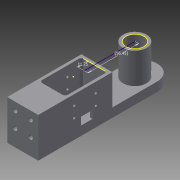
# Autodesk Inventor part: JointBase
Saved by Autodesk Inventor 2015 (Build 190159000, 159)
## iProperties
Created: 2016-04-06
Part Number: JointBase
Material: Generic
Document SubType Name: Modeling
Designer: Hatch
Density: 1 g/cm^3
Appearance: Default
Author: Hatch
Autodesk Inventor part; units mm, degrees
ref_plane "YZ Plane" through (0, 0, 0) normal (1, 0, 0) x (0, 1, 0)
ref_plane "XZ Plane" through (0, 0, 0) normal (0, 1, 0) x (-1, 0, 0)
ref_plane "XY Plane" through (0, 0, 0) normal (0, 0, 1) x (1, 0, 0)
sketch "Sketch1" plane through (0, 0, 0) normal (0, 1, 0) x (-1, 0, 0)
  line L0 (-17.25, 26.25) -> (17.25, 26.25)
  line L1 (17.25, 26.25) -> (17.25, -26.25)
  line L2 (17.25, -26.25) -> (-17.25, -26.25)
  line L3 (-17.25, -26.25) -> (-17.25, 26.25)
  line L4 (-17.25, 26.25) -> (17.25, -26.25) construction
  line L5 (17.25, 26.25) -> (-17.25, -26.25) construction
  line L6 (17.25, -26.25) -> (-17.25, -26.25)
  line L7 (-17.25, -26.25) -> (-17.25, -76.25)
  line L8 (-17.25, -76.25) -> (17.25, -76.25)
  line L9 (17.25, -76.25) -> (17.25, -26.25)
  arc A0 (-17.25, -76.25) -> (17.25, -76.25) centre (0, -76.25) ccw
  point P0 (0, 0)
  dimension "d0" = 34.5
  dimension "d1" = 52.5
  dimension "d4" = 50
  constraints: 20 end point, 4 parallel, 3 midpoint, 2 horizontal, 2 perpendicular, 2 point on circle, 1 centre point
  measures "d0" distance of L1.end L2.end
  measures "d1" distance of L0.end L1.end
  measures "d4" distance of L7.end L6.end
extrude "Floor" add sketch "Sketch1" along normal blind 10
sketch "Sketch3" plane through (0, 10, 0) normal (0, 1, 0) x (1, 0, 0)
  arc A0 (17.25, 76.25) -> (-17.25, 76.25) centre (0, 76.25) ccw
  circle A1 centre (0, 68.45) radius 10
  circle A2 centre (0, 68.45) radius 13
  line L0 (14.25, -23.25) -> (-14.25, -23.25)
  line L1 (-14.25, -23.25) -> (-14.25, 23.25)
  line L2 (-14.25, 23.25) -> (14.25, 23.25)
  line L3 (14.25, 23.25) -> (14.25, -23.25)
  line L4 (14.25, -23.25) -> (-14.25, 23.25) construction
  line L5 (-14.25, -23.25) -> (14.25, 23.25) construction
  line L6 (17.25, 26.25) -> (-17.25, 26.25)
  line L7 (-17.25, 26.25) -> (-17.25, -26.25)
  line L8 (-17.25, -26.25) -> (17.25, -26.25)
  line L9 (17.25, -26.25) -> (17.25, 26.25)
  line L10 (17.25, 26.25) -> (-17.25, -26.25) construction
  line L11 (-17.25, 26.25) -> (17.25, -26.25) construction
  line L12 (0, 23.25) -> (0, 68.45)
  point P0 (0, 0)
  dimension "d14" = 20
  dimension "d18" = 28.5
  dimension "d19" = 46.5
  dimension "d38" = 45.2
  dimension "d54" = 26
  constraints: 26 end point, 5 midpoint, 4 parallel, 3 centre point, 2 coincident, 2 horizontal, 2 perpendicular, 2 point on circle, 1 vertical
  measures "d14" diameter of A1
  measures "d18" distance of L1.end L2.end
  measures "d19" distance of L0.end L1.end
  measures "d38" distance of L12.start L12.end
  measures "d54" diameter of A2
extrude "Slots" add sketch "Sketch3" along normal blind 34
sketch "Sketch4" plane through (17.25, 0, 26.25) normal (1, 0, 0) x (0, 0, -1)
  line L0 (3, 10) -> (49.5, 10)
  line L1 (49.5, 10) -> (49.5, 44)
  line L2 (49.5, 44) -> (3, 44)
  line L3 (3, 44) -> (3, 10)
  line L4 (26.25, 10) -> (38.25, 10)
  line L5 (3, 10) -> (49.5, 10) projected
  line L6 (38.25, 10) -> (14.25, 10)
  line L7 (10.25, 33) -> (34.25, 33)
  line L8 (34.25, 33) -> (34.25, 21)
  line L9 (34.25, 21) -> (10.25, 21)
  line L10 (10.25, 21) -> (10.25, 33)
  line L11 (10.25, 33) -> (34.25, 21) construction
  line L12 (34.25, 33) -> (10.25, 21) construction
  circle A0 centre (10.25, 33) radius 1.35
  circle A1 centre (34.25, 33) radius 1.35
  circle A2 centre (34.25, 21) radius 1.35
  circle A3 centre (10.25, 21) radius 1.35
  line L13 (49.5, 10) -> (49.5, 44) projected
  line L14 (49.5, 27) -> (34.25, 27)
  line L15 (34.25, 27) -> (22.25, 27)
  point P0 (26.25, 0)
  point P1 (22.25, 27)
  dimension "d0" = 34.5
  dimension "d24" = 12
  dimension "d25" = 24
  dimension "d26" = 2.7
  dimension "d27" = 2.7
  dimension "d28" = 2.7
  dimension "d29" = 2.7
  dimension "d56" = 15.25
  dimension "d57" = 12
  constraints: 28 end point, 5 midpoint, 4 centre point, 4 coincident, 4 parallel, 3 perpendicular, 2 horizontal, 2 point on line
  measures "d24" distance of L7.end L8.end
  measures "d25" distance of L8.end L9.end
  measures "d26" diameter of A0
  measures "d27" diameter of A1
  measures "d28" diameter of A2
  measures "d29" diameter of A3
  measures "d56" distance of L14.start L14.end
  measures "d57" distance of L15.end L14.end
extrude "Screws/Sides" cut sketch "Sketch4" against normal through all contours A1 L7 L8 | L8 L7 A1 | A2 L9 L8 | L8 L9 A2 | A0 L10 L7 | L7 L10 A0 | A3 L10 L9 | L9 L10 A3
sketch "Sketch5" plane through (0, 44, 0) normal (0, 1, 0) x (1, 0, 0)
  line L0 (14.25, -21.25) -> (-14.25, -21.25)
  line L1 (-14.25, -21.25) -> (-14.25, 21.25)
  line L2 (-14.25, 21.25) -> (14.25, 21.25)
  line L3 (14.25, 21.25) -> (14.25, -21.25)
  line L4 (14.25, -21.25) -> (-14.25, 21.25) construction
  line L5 (-14.25, -21.25) -> (14.25, 21.25) construction
  line L6 (12.25, 23.25) -> (-12.25, 23.25)
  line L7 (-12.25, 23.25) -> (-12.25, -23.25)
  line L8 (-12.25, -23.25) -> (12.25, -23.25)
  line L9 (12.25, -23.25) -> (12.25, 23.25)
  line L10 (12.25, 23.25) -> (-12.25, -23.25) construction
  line L11 (-12.25, 23.25) -> (12.25, -23.25) construction
  line L12 (-12.25, 21.25) -> (-14.25, 21.25)
  line L13 (12.25, 23.25) -> (12.25, 21.25)
  line L14 (12.25, -21.25) -> (14.25, -21.25)
  line L15 (12.25, -23.25) -> (12.25, -21.25)
  line L16 (-14.25, -21.25) -> (-14.25, -23.25)
  line L17 (-14.25, -23.25) -> (-12.25, -23.25)
  line L18 (-14.25, -21.25) -> (-12.25, -23.25)
  line L19 (-14.25, -23.25) -> (-14.25, -21.25)
  line L20 (-14.25, 21.25) -> (-12.25, 23.25)
  line L21 (-14.25, 23.25) -> (-14.25, 21.25)
  line L22 (-14.25, -23.25) -> (-14.25, 23.25) projected
  line L23 (12.25, 23.25) -> (14.25, 23.25)
  line L24 (14.25, 23.25) -> (14.25, 21.25)
  line L25 (12.25, 23.25) -> (14.25, 21.25)
  line L26 (14.25, 23.25) -> (12.25, 23.25)
  line L27 (14.25, -23.25) -> (12.25, -23.25)
  line L28 (14.25, -23.25) -> (-14.25, -23.25) projected
  line L29 (14.25, -21.25) -> (12.25, -23.25)
  line L30 (14.25, -23.25) -> (14.25, -21.25)
  line L31 (14.25, 23.25) -> (14.25, -23.25) projected
  line L32 (-14.25, 23.25) -> (-12.25, 23.25)
  line L33 (14.25, 23.25) -> (-14.25, 23.25) projected
  point P0 (0, 0)
  dimension "d32" = 42.5
  dimension "d33" = 24.5
  constraints: 60 end point, 7 collinear, 6 point on line, 5 perpendicular, 4 midpoint, 4 parallel, 3 horizontal, 1 vertical
  measures "d32" distance of L0.end L1.end
  measures "d33" distance of L8.end L7.end
extrude "Servo Corners" add sketch "Sketch5" against normal blind 34 contours L30 L27 L29 | L25 L23 L24 | L17 L16 L18 | L20 L21 L32
sketch "Sketch6" plane through (0, 44, 0) normal (0, 1, 0) x (1, 0, 0)
  line L0 (-12.25, 23.25) -> (12.25, 23.25) projected
  line L1 (0, 23.25) -> (0, 12)
  circle A0 centre (0, 68.45) radius 10 projected
  line L2 (0, 12) -> (0, 68.45)
  point P0 (0, 0)
  dimension "d36" = 11.25
  dimension "d37" = 56.45
  constraints: 4 end point, 2 vertical, 1 midpoint
  measures "d36" distance of L1.start L1.end
  measures "d37" distance of L1.end L2.end
sketch "Sketch7" plane through (-17.25, 0, 26.25) normal (0, 0, 1) x (1, 0, 0)
  line L0 (0, 0) -> (34.5, 0)
  line L1 (34.5, 0) -> (34.5, 44)
  line L2 (34.5, 44) -> (0, 44)
  line L3 (0, 44) -> (0, 0)
  point P0 (17.25, 0)
  constraints: 8 end point, 2 parallel, 1 horizontal, 1 perpendicular
extrude "Mount Extension" add sketch "Sketch7" along normal blind 30
sketch "Sketch8" plane through (-17.25, 0, 56.25) normal (0, 0, 1) x (1, 0, 0)
  line L0 (17.25, 0) -> (17.25, 10)
  line L1 (29.5, 44) -> (5, 44) projected
  line L2 (17.25, 27) -> (17.25, 35.5)
  line L3 (34.5, 10) -> (34.5, 44) projected
  line L4 (0, 10) -> (0, 44) projected
  line L5 (17.25, 35.5) -> (8.625, 35.5)
  circle A0 centre (8.625, 35.5) radius 2.6035
  line L6 (17.25, 10) -> (8.625, 10)
  line L7 (29.5, 10) -> (5, 10) projected
  line L8 (8.625, 10) -> (8.625, 18.5)
  circle A1 centre (8.625, 18.5) radius 2.6035
  line L9 (34.5, 35.5) -> (25.875, 35.5)
  dimension "d41" = 10
  dimension "d42" = 5.207
  dimension "d43" = 8.5
  dimension "d44" = 5.207
  dimension "d47" = 8.625
  constraints: 12 end point, 2 centre point, 2 coincident, 2 point on line, 1 horizontal, 1 perpendicular, 1 vertical
  measures "d41" distance of L0.start L0.end
  measures "d42" diameter of A0
  measures "d43" distance of L6.end L8.end
  measures "d44" diameter of A1
  measures "d47" distance of L9.start L9.end
extrude "Mount Holes" cut sketch "Sketch8" against normal blind 20
pattern_linear "Rectangular Pattern1" count 2 spacing 17.25 along (1, 0, 0) of "Mount Holes"
sketch "Sketch11" plane through (17.25, 0, -76.25) normal (1, 0, 0) x (0, 0, -1)
  line L0 (-85.05, 10) -> (-72.05, 10)
  line L1 (-72.05, 10) -> (-72.05, 18.5)
  line L2 (-72.05, 18.5) -> (-85.05, 18.5)
  line L3 (-85.05, 18.5) -> (-85.05, 10)
  circle A0 centre (-68.25, 21) radius 1.35 projected
  line L4 (-68.25, 21) -> (-68.25, 10)
  line L5 (-97.5, 10) -> (-55, 10) projected
  line L6 (-68.25, 10) -> (-72.05, 10)
  point P0 (-76.25, 0)
  dimension "d58" = 13
  dimension "d59" = 8.5
  dimension "d60" = 3.8
  constraints: 12 end point, 2 parallel, 2 point on line, 1 horizontal, 1 perpendicular, 1 vertical
  measures "d58" distance of L2.end L1.end
  measures "d59" distance of L0.end L1.end
  measures "d60" distance of L4.end L0.end
extrude "Wiring Holes" cut sketch "Sketch11" against normal through all contours L3 L2 L1 L0
body "Solid3"
